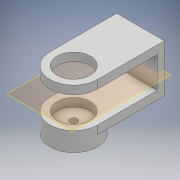
# Autodesk Inventor part: baseRotor1
Saved by Autodesk Inventor 2017 (Build 210142000, 142)
## iProperties
Created: 2017-08-06
Part Number: baseRotor1
Material: Generic
Document SubType Name: Sheet Metal
Designer: Bardo91
Density: 1 g/cm^3
Sheet Metal Rule: Default_mm
Appearance: Default
Author: Bardo91
Autodesk Inventor part; units mm, degrees
ref_plane "YZ Plane" through (0, 0, 0) normal (1, 0, 0) x (0, 1, 0)
ref_plane "XZ Plane" through (0, 0, 0) normal (0, 1, 0) x (-1, 0, 0)
ref_plane "XY Plane" through (0, 0, 0) normal (0, 0, 1) x (1, 0, 0)
sketch "Sketch1" plane through (0, 0, 0) normal (0, 0, 1) x (1, 0, 0)
  circle A0 centre (0, 0) radius 14
  circle A1 centre (0, 0) radius 20
  line L0 (-20, 0) -> (-20, 50)
  line L1 (-20, 50) -> (20, 50)
  line L2 (20, 50) -> (20, 0)
  dimension "d0" = 28
  dimension "d1" = 40
  dimension "d2" = 50
  dimension "d3" = 40
  constraints: 6 end point, 2 centre point, 2 coincident, 2 perpendicular, 2 point on circle, 1 vertical
  measures "d0" diameter of A0
  measures "d1" diameter of A1
  measures "d2" distance of L0.start L0.end
  measures "d3" distance of L0.end L1.end
extrude "Extrusion1" add sketch "Sketch1" along normal blind 7
ref_plane "Work Plane1" through (0, 0, -13) normal (0, 0, 1) x (1, 0, 0)
mirror "Mirror1" about plane through (0, 0, -13) normal (0, 0, 1) of "Extrusion1"
sketch "Sketch2" plane through (0, 0, -33) normal (0, 0, -1) x (-1, 0, 0)
  circle A0 centre (0, 0) radius 14 projected
  circle A1 centre (0, 0) radius 20
  dimension "d11" = 40
  constraints: 1 centre point, 1 coincident
  measures "d11" diameter of A1
extrude "Extrusion2" add sketch "Sketch2" along normal blind 9 contours A0 | A1
sketch "Sketch3" plane through (0, 0, -33) normal (0, 0, 1) x (1, 0, 0)
  circle A0 centre (0, 0) radius 3.1
  dimension "d14" = 6.2
  constraints: 1 centre point, 1 coincident
  measures "d14" diameter of A0
extrude "Extrusion3" cut sketch "Sketch3" against normal blind 1
sketch "Sketch4" plane through (0, 0, -34) normal (0, 0, 1) x (1, 0, 0)
  circle A0 centre (0, 0) radius 3.1
  line L0 (0, 0) -> (0, -1.5)
  line L1 (0, -1.5) -> (-2.7129, -1.5)
  line L2 (0, -1.5) -> (2.7129, -1.5)
  dimension "d17" = 6.2
  dimension "d18" = 1.5
  constraints: 6 end point, 2 horizontal, 2 point on circle, 1 centre point, 1 coincident, 1 vertical
  measures "d17" diameter of A0
  measures "d18" distance of L0.start L0.end
extrude "Extrusion4" cut sketch "Sketch4" against normal through all contours A0 L2 L1 picked at (-0.0193, 1.5513)
sketch "Sketch5" plane through (-20, 50, 0) normal (0, 1, 0) x (1, 0, 0)
  line L0 (0, 0) -> (0, -7) projected
  line L1 (0, 33) -> (40, 33) projected
  line L2 (0, -7) -> (40, -7)
  line L3 (40, -7) -> (40, 33)
  line L4 (40, 33) -> (0, 33)
  line L5 (0, 33) -> (0, -7)
  point P0 (20, 0)
  constraints: 8 end point, 2 parallel, 1 horizontal, 1 perpendicular
extrude "Extrusion5" add sketch "Sketch5" along normal blind 6
equation "\"BendRadius\" = Thickness"
equation "\"BendReliefWidth\" = Thickness"
equation "\"BendReliefDepth\" = 0.5 * Thickness"
equation "\"CornerReliefSize\" = 4 * Thickness"
equation "\"MinimumRemnant\" = 2 * Thickness"
equation "\"TransitionRadius\" = BendRadius"
equation "\"JacobiRadiusSize\" = BendRadius"
equation "\"GapSize\" = Thickness"
equation "\"Thickness\" = 0.5"
body "Solid1"
